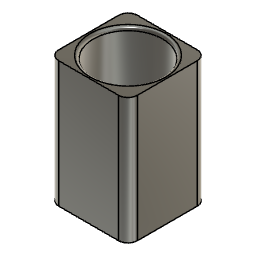
thru hole connector v1 (Autodesk Fusion 360 design; units mm, degrees)
Autodesk Fusion 360 part; units mm, degrees
sketch "Sketch1" plane through (0, 0, 0) normal (0, 0, 1) x (1, 0, 0)
  line L0 (0, 0) -> (-25, 0)
  line L1 (-25, 0) -> (-25, 25)
  line L2 (-25, 25) -> (0, 25)
  line L3 (0, 25) -> (0, 0)
  line L4 (-12.5, 25) -> (-12.5, 0) construction
  line L5 (-25, 12.5) -> (0, 12.5) construction
  circle A0 centre (-12.5, 12.5) radius 11
  circle A1 centre (-12.5, 12.5) radius 10.5
  dimension "d1" = 25
  dimension "d2" = 25
  dimension "d3" = 22
  dimension "d4" = -0.5
  constraint horizontal L0
  constraint vertical L1
  constraint horizontal L2
  constraint vertical L3
  constraint coincident L0.start L3.end
  constraint midpoint L2 L4.start
  constraint midpoint L0 L4.end
  constraint midpoint L1 L5.start
  constraint midpoint L3 L5.end
  constraint midpoint L4 A0.centre
  measures "d1" distance of L0.start L0.end
  measures "d2" distance of L0.start L2.end
  measures "d3" diameter of A0
extrude "Extrude1" add sketch "Sketch1" along normal mid plane 2 draft -45 contours A0 makes body 1
extrude "Extrude2" add sketch "Sketch1" along normal mid plane 40 separate body contours L0 L1 L2 L3 makes body 2
fillet "Fillet1" radius 1 1 edges at (-22.7556, 16.4778, 20) on bodies 2
fillet "Fillet2" radius 1 1 edges at (-22.7556, 8.5222, -20) on bodies 2
fillet "Fillet3" radius 3 4 edges at (-25, 25, 0) (0, 25, 0) (0, 0, 0) (-25, 0, 0) on bodies 2
